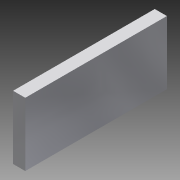
# Autodesk Inventor part: CavitySplitter
Saved by Autodesk Inventor 2014 (Build 180170000, 170)
## iProperties
Created: 2015-04-19
Part Number: CavitySplitter
Material: Generic
Document SubType Name: Modeling
Designer: Owner
Density: 1 g/cm^3
Appearance: Aluminum - Polished
Author: Owner
Autodesk Inventor part; units mm, degrees
ref_plane "YZ Plane" through (0, 0, 0) normal (1, 0, 0) x (0, 1, 0)
ref_plane "XZ Plane" through (0, 0, 0) normal (0, 1, 0) x (-1, 0, 0)
ref_plane "XY Plane" through (0, 0, 0) normal (0, 0, 1) x (1, 0, 0)
sketch "Sketch1" plane through (0, 0, 0) normal (1, 0, 0) x (0, 1, 0)
  line L0 (-65.0537, 22.225) -> (-7.9037, 22.225)
  line L1 (-7.9037, 22.225) -> (-7.9037, -22.225)
  line L2 (-7.9037, -22.225) -> (-65.0537, -22.225)
  line L3 (-65.0537, -22.225) -> (-65.0537, 22.225)
  line L4 (-7.9037, -3.175) -> (-23.1437, -3.175)
  line L5 (-23.1437, -3.175) -> (-23.1437, 9.525)
  line L6 (-23.1437, 9.525) -> (-7.9037, 9.525)
  line L7 (-7.9037, 9.525) -> (-7.9037, -3.175)
  line L8 (-7.9037, -22.225) -> (-46.0037, -22.225)
  line L9 (-46.0037, -22.225) -> (-46.0037, -32.385)
  line L10 (-46.0037, -32.385) -> (-7.9037, -32.385)
  line L11 (-7.9037, -32.385) -> (-7.9037, -22.225)
  point P0 (0, 0)
  dimension "d2" = 57.15
  dimension "d3" = 44.45
  dimension "d4" = 15.24
  dimension "d5" = 12.7
  dimension "d7" = 10.16
  dimension "d8" = 38.1
  dimension "d10" = 19.05
  constraints: 24 end point, 6 parallel, 3 horizontal, 3 perpendicular, 1 point on line
  measures "d2" distance of L0.start L0.end
  measures "d3" distance of L0.end L1.end
  measures "d4" distance of L5.end L6.end
  measures "d5" distance of L4.end L5.end
  measures "d7" distance of L10.end L1.end
  measures "d8" distance of L9.end L10.end
  measures "d10" distance between parallel lines of L2 L4
extrude "Extrusion1" add sketch "Sketch1" along normal blind 6.35 contours L0 L1 L6 L5 L4 L2 L3 | L2 L11 L10 L9
body "Solid1"
